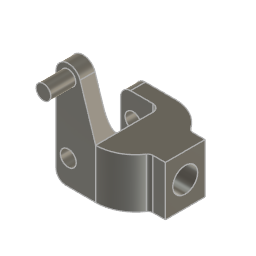
steering_mechanism (Autodesk Fusion 360 archive; units mm, degrees)
design "front wheel mount"
Autodesk Fusion 360 part; units mm, degrees
sketch "Sketch1" plane through (0, 0, 0) normal (0, 0, 1) x (1, 0, 0)
  line L0 (-31, 32) -> (-23, 32)
  line L1 (-23, 32) -> (-23, 29)
  line L2 (-23, 29) -> (-31, 29)
  line L3 (-31, 29) -> (-31, 32)
  line L4 (-31, 19) -> (-23, 19)
  line L5 (-23, 19) -> (-23, 16)
  line L6 (-23, 16) -> (-31, 16)
  line L7 (-31, 16) -> (-31, 19)
  line L8 (-23, 19) -> (-23, 29)
  arc A0 (-23, 19) -> (-23, 29) centre (-23, 24) ccw
  arc A1 (-23, 16) -> (-23, 32) centre (-23, 24) ccw
  line L9 (-23, 20) -> (-13, 20)
  line L10 (-13, 20) -> (-13, 28)
  line L11 (-13, 28) -> (-23, 28)
  line L12 (-23, 28) -> (-23, 20)
  dimension "d1" = 8
  dimension "d2" = 3
  dimension "d15" = 10
  dimension "d16" = 10
  dimension "d17" = 8
  constraint horizontal L0
  constraint vertical L1
  constraint horizontal L2
  constraint vertical L3
  constraint horizontal L4
  constraint vertical L5
  constraint horizontal L6
  constraint vertical L7
  constraint collinear L3 L7
  constraint equal L3 L7
  constraint equal L2 L4
  constraint midpoint L8 A0.centre
  constraint concentric A0 A1
  constraint horizontal L9
  constraint vertical L10
  constraint horizontal L11
  constraint vertical L12
  constraint coincident L8 L9.start
  constraint midpoint L8 L12
  measures "d1" distance of L0.start L0.end
  measures "d2" distance of L0.start L2.end
  measures "d15" distance of L2 L4
  measures "d16" distance of L9.start L9.end
  measures "d17" distance of L9.start L11.end
  measures "d88" diameter of A0.centre
extrude "Extrude1" add sketch "Sketch1" along normal blind 10
hole "Hole1" at (-13, 24, 5) direction (-1, 0, 0) diameter 5 end through all
sketch "Sketch2" plane through (0, 32, 0) normal (0, 1, 0) x (-1, 0, 0)
  line L0 (23, 0) -> (31, 0)
  line L1 (31, 0) -> (31, 10)
  line L2 (31, 10) -> (23, 10)
  circle A0 centre (28.5, 5) radius 1.6
  line L3 (23, 10) -> (23, 0)
  line L4 (28.5, 10) -> (28.5, 0) construction
  dimension "d14" = 3.2
  dimension "d55" = 2.5
  constraint coincident L2 L4.start
  constraint coincident L0 L4.end
  constraint perpendicular L0 L4
  constraint midpoint A0.centre L4
  measures "d14" diameter of A0
  measures "d55" distance of L1 A0.centre
sketch "Sketch3" plane through (0, 0, 10) normal (0, 0, 1) x (-1, 0, 0)
  line L0 (23, -29) -> (23, -19)
  line L1 (23, -19) -> (31, -19)
  line L2 (31, -19) -> (31, -16)
  line L3 (31, -16) -> (23, -16)
  arc A0 (23, -16) -> (16.0718, -20) centre (23, -24) ccw
  line L4 (13, -20) -> (13, -28)
  line L5 (13, -28) -> (16.0718, -28)
  arc A1 (16.0718, -28) -> (23, -32) centre (23, -24) ccw
  line L6 (23, -32) -> (31, -32)
  line L7 (31, -32) -> (31, -29)
  line L8 (31, -29) -> (23, -29)
  line L9 (31, -16) -> (23, -16)
  line L10 (23, -16) -> (23, -19)
  line L11 (23, -19) -> (31, -19)
  line L12 (31, -19) -> (31, -16)
  line L13 (16.0718, -20) -> (13, -20)
  constraint horizontal L9
  constraint vertical L10
  constraint horizontal L11
  constraint vertical L12
  constraint coincident L2.end L3.start
  constraint collinear L1 L11
  constraint collinear L0 L10
extrude "Extrude2" add sketch "Sketch3" along normal blind 14 contours L1 L2 L3 L9 L10 L11 L12
extrude "Extrude4" cut sketch "Sketch2" against normal through all contours A0
sketch "Sketch6" plane through (0, 16, 0) normal (0, -1, 0) x (1, 0, 0)
  line L0 (-31, 24) -> (-31, 0)
  line L1 (-31, 0) -> (-23, 0)
  line L2 (-23, 0) -> (-23, 10)
  line L3 (-28.5, 5) -> (-28.5, 19) construction
  circle A0 centre (-28.5, 19) radius 1.5
  circle A1 centre (-28.5, 5) radius 1.6
  line L4 (-23, 10) -> (-23, 24)
  line L5 (-23, 24) -> (-31, 24)
  point P0 (-28.5, 5)
  dimension "d50" = 14
  dimension "d51" = 3
  constraint vertical L3
  constraint coincident L3.end A0.centre
  constraint coincident P0 L3.start
  measures "d50" distance of P0 L3.end
  measures "d51" diameter of A0
extrude "Extrude6" add sketch "Sketch6" along normal blind 5 contours A0
move_face "OffsetFaces1" offset 5 1 faces at (-31, 17, 16)
sketch "Sketch4" plane through (0, 16, 0) normal (0, 1, 0) x (-1, 0, 0)
  circle A0 centre (28.5, 3) radius 1.5
  line L0 (23, 0) -> (36, 0)
  line L1 (36, 0) -> (36, 24)
  line L2 (36, 24) -> (23, 24)
  line L3 (23, 24) -> (23, 10)
  line L4 (23, 10) -> (23, 0)
  line L5 (31, 19) -> (31, 0)
  circle A1 centre (28.5, 3) radius 2.5 construction
  line L6 (23, 10) -> (26.1186, 19.7609)
  circle A2 centre (28.5, 5) radius 1.6
  circle A3 centre (28.5, 5) radius 1.6
  circle A4 centre (28.5, 19) radius 1.5
  circle A5 centre (28.5, 19) radius 2.5
  dimension "d73" = 1
  dimension "d88" = 5
  constraint vertical L5
  constraint coincident L0 L5.end
  constraint tangent L5 A1
  constraint coincident L3.end L4.start
  constraint concentric A4 A5
  constraint coincident L5.start A5
  constraint coincident L6.end A5
  constraint tangent L6 A5
  measures "d88" diameter of A5
extrude "Extrude7" cut sketch "Sketch4" along normal up to surface (3 mm away) contours L0 L1 L2 L3 L5 L6 A5
fillet "Fillet2" radius 1 2 edges at (-16.0718, 20, 5) (-16.0718, 28, 5)
fillet "Fillet6" radius 2 3 edges at (-31, 17.5, 0) (-31, 30.5, 0) (-31, 30.5, 10)
fillet "Fillet7" radius 1.5 2 edges at (-23, 19, 5) (-23, 29, 5)
move_face "OffsetFaces2" [suppressed]
sketch "Sketch7" plane through (-23, 0, 0) normal (-1, 0, 0) x (0, -1, 0)
  circle A0 centre (-24, 5) radius 2.5
  line L0 (-27.5, 0) -> (-20.5, 0)
  line L1 (-20.5, 10) -> (-27.5, 10)
  circle A1 centre (-24, 5) radius 3.875
  line L2 (-27.5, 10) -> (-27.5, 0)
  line L3 (-20.5, 0) -> (-20.5, 10)
  dimension "d81" = 7.75
  constraint concentric A0 A1
  measures "d81" diameter of A1
extrude "Extrude8" cut sketch "Sketch7" against normal blind 4 contours A1 L2 L3 | A1 L2 | A1 L3
extrude "Extrude10" cut 2 faces at (-23, 20.4311, 5.3764) (-23, 27.5689, 5.3764) along direction (-1, 0, 0) blind 1
named bodies: "front wheel mount"
